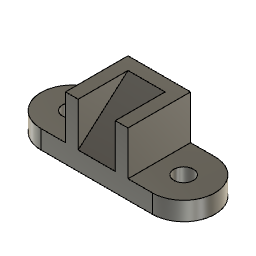
A2 (Autodesk Fusion 360 design; units mm, degrees)
Autodesk Fusion 360 part; units mm, degrees
sketch "Sketch1" plane through (0, 0, 0) normal (0, 0, 1) x (1, 0, 0)
  line L0 (57, 32) -> (-57, 32)
  line L1 (-57, -32) -> (57, -32)
  circle A0 centre (57, 0) radius 10
  circle A1 centre (-57, 0) radius 10
  arc A2 (29.6806, -16.6628) -> (30.3525, -17.7176) centre (57, 0) ccw
  arc A3 (57, -32) -> (57, 32) centre (57, 0) ccw
  arc A4 (30.3525, 17.7176) -> (29.6806, 16.6628) centre (57, 0) ccw
  line L2 (30.3525, 17.04) -> (29.6806, 16.6628) construction
  line L3 (-29.6806, -16.6628) -> (-30.5407, -17.1456) construction
  line L4 (30.3525, 17.7176) -> (30.3525, 17.04) construction
  line L5 (30.3525, -17.04) -> (30.3525, -17.7176) construction
  line L6 (-30.5407, 17.1456) -> (-29.6806, 16.6628) construction
  line L7 (29.6806, -16.6628) -> (30.3525, -17.04) construction
  line L8 (-30.5407, 17.9973) -> (-30.5407, 17.1456) construction
  line L9 (-30.5407, -17.1456) -> (-30.5407, -17.9973) construction
  arc A5 (-57, 32) -> (-57, -32) centre (-57, 0) ccw
  arc A6 (-30.5407, -17.9973) -> (-29.6806, -16.6628) centre (-57, 0) ccw
  dimension "d1" = 114
  dimension "d2" = 64
  dimension "d3" = 64
  dimension "d4" = 64
  constraint horizontal L0
  constraint parallel L0 L1
  constraint coincident origin L2
  constraint coincident origin L6
  constraint perpendicular L1 L8
  constraint perpendicular L1 L4
  constraint coincident A2.end L4
  constraint coincident A2.start L6
  constraint concentric A2 A3
  constraint concentric A3 A4
  constraint collinear L2 L3
  constraint coincident L5.start L6
  constraint collinear L4 L5
  constraint collinear L6 L7
  constraint collinear L8 L9
  constraint coincident L9.end A5
  constraint concentric A5 A6
  measures "d1" distance of L1.start L1.end
  measures "d2" distance of L0.end L1.start
  measures "d3" diameter of A3
  measures "d4" diameter of A5
extrude "Extrude1" add sketch "Sketch1" along normal blind 19
sketch "Sketch2" plane through (0, 0, 19) normal (0, 0, 1) x (-1, 0, 0)
  circle A0 centre (-57, 0) radius 10
  circle A1 centre (57, 0) radius 10
  arc A2 (57, -32) -> (57, 32) centre (57, 0) ccw
  line L0 (57, 32) -> (-57, 32)
  arc A3 (-57, 32) -> (-57, -32) centre (-57, 0) ccw
  line L1 (-57, -32) -> (57, -32)
  line L2 (32, -32) -> (-32, -32)
  line L3 (-32, -32) -> (-32, 32)
  line L4 (32, 32) -> (32, -32)
  line L5 (19, -19) -> (-19, -19)
  line L6 (-19, -19) -> (-19, 32)
  line L7 (19, 32) -> (19, -19)
  line L8 (-32, 32) -> (-19, 32)
  line L9 (19, 32) -> (32, 32)
  dimension "d9" = 64
  dimension "d11" = 38
  dimension "d12" = 51
  dimension "d13" = 13
  constraint horizontal L2
  constraint vertical L3
  constraint horizontal L8
  constraint vertical L4
  constraint coincident L0 L3.end
  constraint coincident L1 L2.start
  constraint horizontal L5
  constraint vertical L6
  constraint vertical L7
  constraint collinear L8 L9
  measures "d9" distance of L2.start L2.end
  measures "d11" distance of L5.start L5.end
  measures "d12" distance of L5.start L7.start
  measures "d13" distance of L4 L7
extrude "Extrude2" add sketch "Sketch2" along normal blind 45 contours L0 L1 L2 L3 L4 L5 L6 L7 L8 L9
sketch "Sketch3" plane through (0, 0, 0) normal (1, 0, 0) x (0, 1, 0)
  line L0 (19, 63.9719, -30) -> (19, 18.9719, -30)
  line L1 (19, 18.9719, -30) -> (-32, 18.9719, -30)
  line L2 (-32, 18.9719, -30) -> (19, 63.9719, -30)
  dimension "d16" = 45
  dimension "d18" = 51
extrude "Extrude3" add sketch "Sketch3" along normal blind 55 contours L0 L1 L2 in plane through (-30, 0, 0) normal (1, 0, 0)
equation "d14 = 64 mm - 19 mm"
equation "d16 = 64 mm - 19 mm"
